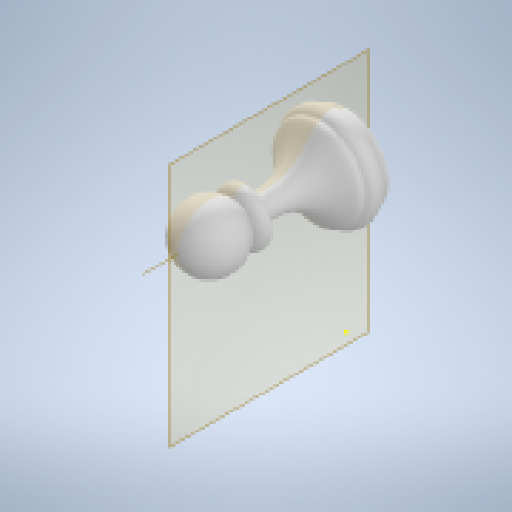
# Autodesk Inventor part: pawn-white-v2
Saved by Autodesk Inventor 2024.1 (Build 281209000, 209)
## iProperties
Created: 2025-08-03
Part Number: pawn-white-v2
Material: Generic
Document SubType Name: Modeling
Designer: iwheard
Density: 1 g/cm^3
Appearance: Default
Author: iwheard
Autodesk Inventor part; units mm, degrees
(part 1 of 2)
ref_plane "XZ Plane" through (0, 0, 0) normal (0, 1, 0) x (-1, 0, 0)
ref_plane "XY Plane" through (0, 0, 0) normal (0, 0, 1) x (1, 0, 0)
sketch "Sketch1" plane through (0, 0, 0) normal (0, 0, 1) x (1, 0, 0)
  circle A0 centre (0, 25.5) radius 3
  circle A1 centre (0, 25.5) radius 5
  point P0 (0, 0)
  dimension "d0" = 10
  constraints: 2 centre point
  measures "d0" diameter of A1
extrude "Extrusion1" add sketch "Sketch1" along normal blind 3
sketch "Sketch3" plane through (0, 25.5, 3) normal (0, 0, 1) x (1, 0, 0)
  circle A0 centre (0, 0) radius 5 projected
  circle A1 centre (0, 0) radius 3 projected
  circle A2 centre (0, 0) radius 7.15
  point P0 (0, -25.5)
  dimension "d6" = 14.3
  constraints: 1 centre point
  measures "d6" diameter of A2
extrude "Extrusion2" add sketch "Sketch3" against normal blind 3 contours A2
sketch "Sketch2" plane through (0, 0, 0) normal (1, 0, 0) x (0, 1, 0)
  line L0 (30.5, 3) -> (20.5, 3) projected
  circle A0 centre (25.5, 23) radius 5.25
  line L1 (30.5, 0) -> (20.5, 0) projected
  line L2 (25.5, 28.25) -> (25.5, 3)
  line L3 (28.7742, 18.8961) -> (28.7225, 18.9815) construction
  line L4 (27.5353, 15.1585) -> (27.5353, 12.8331) construction
  line L5 (27.5353, 12.8331) -> (27.8628, 9.8109) construction
  line L6 (27.8628, 9.8109) -> (30.696, 6.4585) construction
  line L7 (30.696, 6.4585) -> (33.4932, 5.0528) construction
  line L8 (34.1113, 1.8552) -> (32.8751, 0.9289) construction
  line L9 (32.8751, 0.9289) -> (32.65, 0.7147) construction
  spline S0 degree 4 poles (28.7742, 18.8961) (28.7225, 18.9815) (30.0018, 18.4917) (30.1859, 16.8801) (29.2697, 16.5797) (27.9179, 16.8801) (27.9179, 16.1364) (27.5353, 15.1585) (27.5353, 12.8331) (27.8628, 9.8109) (30.696, 6.4585) (33.4932, 5.0528) (32.5369, 4.2802) (33.817, 3.9218) (34.1113, 1.8552) (32.8751, 0.9289) (32.65, 0.7147) knots 0 0 0 0 0 0.002456 0.076412 0.193262 1 2 3 4 5 6 7 7.40272 8 9 9 9 9 9
  line L10 (30.5, 0) -> (30.5, 3) projected
  line L11 (27.9179, 16.1364) -> (27.5353, 15.1585) construction
  line L12 (28.5, 3) -> (28.5, 0) projected
  line L13 (32.65, 3) -> (18.35, 3) projected
  line L14 (32.65, 3) -> (32.65, 0) projected
  line L15 (33.4932, 5.0528) -> (32.5369, 4.2802) construction
  line L16 (32.5369, 4.2802) -> (33.817, 3.9218) construction
  line L17 (33.817, 3.9218) -> (34.1113, 1.8552) construction
  line L18 (27.9179, 16.8801) -> (27.9179, 16.1364) construction
  line L19 (29.2697, 16.5797) -> (27.9179, 16.8801) construction
  line L20 (28.7225, 18.9815) -> (30.0018, 18.4917) construction
  line L21 (30.0018, 18.4917) -> (30.1859, 16.8801) construction
  line L22 (30.1859, 16.8801) -> (29.2697, 16.5797) construction
  point P0 (0, 0)
  point P1 (25.5, 3)
  point P2 (30.5, 0.7117)
  point P3 (28.8281, 18.9396)
  point P4 (25.5, 17.75)
  point P5 (32.65, 0.7147)
  dimension "d3" = 10.5
  dimension "d4" = 23
  constraints: 2 end point, 2 point on circle, 2 vertical alignment, 1 centre point, 1 midpoint, 4 other
  measures "d3" diameter of A0
  measures "d4" distance from line of L1 A0.centre
revolve "Revolution1" add sketch "Sketch2" angle 360 about axis through (0, 25.5, 28.25) along (0, 0, -1) contours L0 L2 A0 S0 L14 L13 | L2 A0 S0 | A0 S0
chamfer "Chamfer1" distance 0.5 angle 45 2 edges at (5.0558, 30.5558, 0.7147) (-5.0558, 20.4442, 0.7147)
sketch "Sketch11" plane through (0, 0, 0) normal (1, 0, 0) x (0, 1, 0)
  line L0 (27.9316, 16.5405) -> (27.8538, 16.3314)
  line L1 (27.8538, 16.3314) -> (28.5086, 16.0877)
  line L2 (28.5086, 16.0877) -> (28.5864, 16.2967)
  line L3 (28.5864, 16.2967) -> (27.9316, 16.5405)
  line L4 (27.837, 16.2536) -> (27.7455, 15.9057)
  line L5 (27.7455, 15.9057) -> (28.4076, 15.7315)
  line L6 (28.4076, 15.7315) -> (28.4991, 16.0794)
  line L7 (28.4991, 16.0794) -> (27.837, 16.2536)
  line L8 (27.7341, 15.8623) -> (27.561, 15.0978)
  line L9 (27.561, 15.0978) -> (28.3711, 14.9144)
  line L10 (28.3711, 14.9144) -> (28.5442, 15.6789)
  line L11 (28.5442, 15.6789) -> (27.7341, 15.8623)
  line L12 (27.5469, 14.9814) -> (27.5027, 14.0719)
  line L13 (27.5027, 14.0719) -> (28.4029, 14.0282)
  line L14 (28.4029, 14.0282) -> (28.4471, 14.9377)
  line L15 (28.4471, 14.9377) -> (27.5469, 14.9814)
  line L16 (27.4909, 13.8281) -> (27.532, 12.6551)
  line L17 (27.532, 12.6551) -> (28.8485, 12.7012)
  line L18 (28.8485, 12.7012) -> (28.8074, 13.8742)
  line L19 (28.8074, 13.8742) -> (27.4909, 13.8281)
  line L20 (27.5561, 12.4959) -> (27.7913, 11.1635)
  line L21 (27.7913, 11.1635) -> (29.3083, 11.4312)
  line L22 (29.3083, 11.4312) -> (29.0732, 12.7637)
  line L23 (29.0732, 12.7637) -> (27.5561, 12.4959)
  line L24 (27.837, 10.9041) -> (28.2953, 9.6805)
  line L25 (28.2953, 9.6805) -> (29.8371, 10.2579)
  line L26 (29.8371, 10.2579) -> (29.3789, 11.4815)
  line L27 (29.3789, 11.4815) -> (27.837, 10.9041)
  line L28 (28.4029, 9.3932) -> (29.3083, 8.0791)
  line L29 (29.3083, 8.0791) -> (30.9089, 9.1819)
  line L30 (30.9089, 9.1819) -> (30.0035, 10.496)
  line L31 (30.0035, 10.496) -> (28.4029, 9.3932)
  line L32 (29.7117, 7.6092) -> (31.4159, 6.0425)
  line L33 (31.4159, 6.0425) -> (33.1005, 7.8751)
  line L34 (33.1005, 7.8751) -> (31.3962, 9.4417)
  line L35 (31.3962, 9.4417) -> (29.7117, 7.6092)
  line L36 (29.7556, 7.5688) -> (32.638, 5.3084)
  line L37 (32.638, 5.3084) -> (33.9032, 6.9217)
  line L38 (33.9032, 6.9217) -> (31.0207, 9.1822)
  line L39 (31.0207, 9.1822) -> (29.7556, 7.5688)
  point P0 (0, 0)
  point P1 (28.3771, 14.9411)
  point P2 (28.2195, 14.9487)
  point P3 (28.6874, 12.6956)
  point P4 (28.8477, 12.7239)
  point P5 (29.1875, 11.4099)
  point P6 (29.3043, 11.4536)
  point P7 (29.4446, 10.1109)
  point P8 (29.8004, 10.356)
  constraints: 80 end point, 20 parallel, 10 perpendicular, 6 point on line
extrude "Extrusion6" cut sketch "Sketch11" along normal mid plane 10 contours L3 L2 L1 L0 | L7 L6 L5 L4 | L11 L10 L15 L9 L8 | L15 L10 L9 | L9 L10 L15 L14 L13 L12 | L19 L18 L23 L17 L16 | L17 L18 L23 L22 L27 L21 L20 | L27 L26 L31 L25 L24 L21 L22 | L31 L30 L29 L28 L25 L26 | L35 L39 L32 | L36 L33 L32 | L39 L35 L38 L33 L36 | L39 L38 L35 | L33 L38 L37 L36 | L35 L34 L33 L38
sketch "Sketch12" plane through (-2.1873, 31.7347, 5.7495) normal (0, 0.6767574, 0.7362061) x (1, 0, 0)
  line L0 (14.163, 8.8077) -> (14.3706, 8.3256)
  line L1 (14.3706, 8.3256) -> (14.8236, 7.8122)
  line L2 (14.8236, 7.8122) -> (15.3364, 7.3493)
  line L3 (15.3364, 7.3493) -> (15.9624, 7.2197)
  line L4 (15.9624, 7.2197) -> (16.3471, 7.1936)
  line L5 (16.3471, 7.1936) -> (16.622, 7.2886)
  line L6 (16.622, 7.2886) -> (17.37, 8.2151)
  line L7 (17.37, 8.2151) -> (17.7786, 8.8333)
  line L8 (17.7786, 8.8333) -> (17.8374, 9.0234)
  line L9 (17.8374, 9.0234) -> (17.7788, 9.151)
  line L10 (17.7788, 9.151) -> (17.2482, 9.2679)
  line L11 (17.2482, 9.2679) -> (16.0645, 9.2846)
  line L12 (16.0645, 9.2846) -> (14.2757, 9.225)
  line L13 (14.2757, 9.225) -> (14.099, 9.0834)
  line L14 (14.099, 9.0834) -> (14.163, 8.8077)
  line L15 (-0.827, 7.7393) -> (0.3726, 6.4109)
  line L16 (0.3726, 6.4109) -> (0.6073, 6.298)
  line L17 (0.6073, 6.298) -> (0.8022, 6.3831)
  line L18 (0.8022, 6.3831) -> (1.0932, 6.7181)
  line L19 (1.0932, 6.7181) -> (1.3226, 7.9284)
  line L20 (1.3226, 7.9284) -> (1.4204, 8.7124)
  line L21 (1.4204, 8.7124) -> (1.2832, 9.1151)
  line L22 (1.2832, 9.1151) -> (0.7585, 9.2634)
  line L23 (0.7585, 9.2634) -> (-0.3067, 9.2846)
  line L24 (-0.3067, 9.2846) -> (-1.3546, 9.2605)
  line L25 (-1.3546, 9.2605) -> (-1.758, 9.0914)
  line L26 (-1.758, 9.0914) -> (-1.5659, 8.6327)
  line L27 (-1.5659, 8.6327) -> (-0.827, 7.7393)
  line L28 (7.9724, 8.1152) -> (8.0582, 7.0436)
  line L29 (8.0582, 7.0436) -> (8.456, 6.5585)
  line L30 (8.456, 6.5585) -> (8.9127, 6.2422)
  line L31 (8.9127, 6.2422) -> (9.411, 6.3517)
  line L32 (9.411, 6.3517) -> (9.7063, 6.4776)
  line L33 (9.7063, 6.4776) -> (9.8794, 6.6817)
  line L34 (9.8794, 6.6817) -> (10.1275, 7.9084)
  line L35 (10.1275, 7.9084) -> (10.231, 8.704)
  line L36 (10.231, 8.704) -> (10.1625, 9.1126)
  line L37 (10.1625, 9.1126) -> (9.8294, 9.2631)
  line L38 (9.8294, 9.2631) -> (9.1388, 9.2846)
  line L39 (9.1388, 9.2846) -> (8.4456, 9.2663)
  line L40 (8.4456, 9.2663) -> (8.093, 9.1384)
  line L41 (8.093, 9.1384) -> (7.9717, 8.7913)
  line L42 (7.9717, 8.7913) -> (7.9724, 8.1152)
  line L43 (5.0826, 8.0719) -> (5.1312, 7.3559)
  line L44 (5.1312, 7.3559) -> (5.3208, 6.9613)
  line L45 (5.3208, 6.9613) -> (5.7267, 6.7901)
  line L46 (5.7267, 6.7901) -> (6.4238, 6.744)
  line L47 (6.4238, 6.744) -> (7.4596, 6.7391)
  line L48 (7.4596, 6.7391) -> (7.7676, 6.8351)
  line L49 (7.7676, 6.8351) -> (7.9267, 7.0799)
  line L50 (7.9267, 7.0799) -> (7.9205, 8.1163)
  line L51 (7.9205, 8.1163) -> (7.8791, 8.7917)
  line L52 (7.8791, 8.7917) -> (7.7156, 9.1386)
  line L53 (7.7156, 9.1386) -> (7.295, 9.2663)
  line L54 (7.295, 9.2663) -> (6.4826, 9.2846)
  line L55 (6.4826, 9.2846) -> (5.6709, 9.2657)
  line L56 (5.6709, 9.2657) -> (5.2544, 9.133)
  line L57 (5.2544, 9.133) -> (5.1021, 8.773)
  line L58 (5.1021, 8.773) -> (5.0826, 8.0719)
  line L59 (2.9046, 7.8131) -> (2.9449, 6.9663)
  line L60 (2.9449, 6.9663) -> (3.0705, 6.5566)
  line L61 (3.0705, 6.5566) -> (3.3825, 6.4694)
  line L62 (3.3825, 6.4694) -> (3.982, 6.5898)
  line L63 (3.982, 6.5898) -> (4.5907, 6.7618)
  line L64 (4.5907, 6.7618) -> (4.9028, 6.9733)
  line L65 (4.9028, 6.9733) -> (5.0167, 7.363)
  line L66 (5.0167, 7.363) -> (5.0308, 8.0695)
  line L67 (5.0308, 8.0695) -> (5.0114, 8.772)
  line L68 (5.0114, 8.772) -> (4.8919, 9.1327)
  line L69 (4.8919, 9.1327) -> (4.5702, 9.2656)
  line L70 (4.5702, 9.2656) -> (3.9448, 9.2846)
  line L71 (3.9448, 9.2846) -> (3.3201, 9.2616)
  line L72 (3.3201, 9.2616) -> (3.0035, 9.1007)
  line L73 (3.0035, 9.1007) -> (2.8975, 8.6638)
  line L74 (2.8975, 8.6638) -> (2.9046, 7.8131)
  line L75 (1.9535, 6.3705) -> (2.6599, 6.2006)
  line L76 (2.6599, 6.2006) -> (2.8227, 6.2422)
  line L77 (2.8227, 6.2422) -> (2.8531, 7.8018)
  line L78 (2.8531, 7.8018) -> (2.7404, 9.0993)
  line L79 (2.7404, 9.0993) -> (2.5551, 9.2614)
  line L80 (2.5551, 9.2614) -> (2.2027, 9.2846)
  line L81 (2.2027, 9.2846) -> (1.8475, 9.2634)
  line L82 (1.8475, 9.2634) -> (1.6429, 9.1153)
  line L83 (1.6429, 9.1153) -> (1.3754, 7.9301)
  line L84 (1.3754, 7.9301) -> (1.2613, 7.1439)
  line L85 (1.2613, 7.1439) -> (1.2835, 6.7193)
  line L86 (1.2835, 6.7193) -> (1.4962, 6.5103)
  line L87 (1.4962, 6.5103) -> (1.9535, 6.3705)
  line L88 (10.7348, 6.2426) -> (11.2015, 6.1065)
  line L89 (11.2015, 6.1065) -> (11.5002, 6.2111)
  line L90 (11.5002, 6.2111) -> (11.7035, 6.6792)
  line L91 (11.7035, 6.6792) -> (11.8841, 7.6335)
  line L92 (11.8841, 7.6335) -> (12.0194, 8.588)
  line L93 (12.0194, 8.588) -> (12.0002, 9.0781)
  line L94 (12.0002, 9.0781) -> (11.7686, 9.2588)
  line L95 (11.7686, 9.2588) -> (11.2666, 9.2846)
  line L96 (11.2666, 9.2846) -> (10.7573, 9.2631)
  line L97 (10.7573, 9.2631) -> (10.4744, 9.1124)
  line L98 (10.4744, 9.1124) -> (10.3158, 8.7035)
  line L99 (10.3158, 8.7035) -> (10.1798, 7.9073)
  line L100 (10.1798, 7.9073) -> (10.0695, 7.1065)
  line L101 (10.0695, 7.1065) -> (10.0905, 6.6662)
  line L102 (10.0905, 6.6662) -> (10.2949, 6.4302)
  line L103 (10.2949, 6.4302) -> (10.7348, 6.2426)
  line L104 (16.9589, 6.5843) -> (17.1578, 6.2745)
  line L105 (17.1578, 6.2745) -> (17.393, 6.1023)
  line L106 (17.393, 6.1023) -> (18.5799, 5.9227)
  line L107 (18.5799, 5.9227) -> (19.3386, 5.8753)
  line L108 (19.3386, 5.8753) -> (19.7282, 6.0278)
  line L109 (19.7282, 6.0278) -> (19.8717, 6.5319)
  line L110 (19.8717, 6.5319) -> (19.8922, 7.539)
  line L111 (19.8922, 7.539) -> (19.879, 8.5482)
  line L112 (19.879, 8.5482) -> (19.7863, 9.0664)
  line L113 (19.7863, 9.0664) -> (19.5345, 9.2573)
  line L114 (19.5345, 9.2573) -> (19.0443, 9.2846)
  line L115 (19.0443, 9.2846) -> (18.542, 9.2677)
  line L116 (18.542, 9.2677) -> (18.2057, 9.1491)
  line L117 (18.2057, 9.1491) -> (17.4233, 8.2007)
  line L118 (17.4233, 8.2007) -> (16.7855, 7.1857)
  line L119 (16.7855, 7.1857) -> (16.7926, 6.909)
  line L120 (16.7926, 6.909) -> (16.9589, 6.5843)
  line L121 (12.0155, 5.7626) -> (12.3735, 5.5954)
  line L122 (12.3735, 5.5954) -> (12.8508, 5.6913)
  line L123 (12.8508, 5.6913) -> (13.1456, 5.7916)
  line L124 (13.1456, 5.7916) -> (13.3441, 5.969)
  line L125 (13.3441, 5.969) -> (13.8139, 7.0741)
  line L126 (13.8139, 7.0741) -> (14.2004, 8.2222)
  line L127 (14.2004, 8.2222) -> (14.1104, 8.8011)
  line L128 (14.1104, 8.8011) -> (13.8533, 9.2243)
  line L129 (13.8533, 9.2243) -> (13.0678, 9.2847)
  line L130 (13.0678, 9.2847) -> (12.5587, 9.2588)
  line L131 (12.5587, 9.2588) -> (12.2711, 9.0777)
  line L132 (12.2711, 9.0777) -> (12.0989, 8.5862)
  line L133 (12.0989, 8.5862) -> (11.9359, 7.6291)
  line L134 (11.9359, 7.6291) -> (11.7519, 6.1542)
  line L135 (11.7519, 6.1542) -> (11.824, 5.9105)
  line L136 (11.824, 5.9105) -> (12.0155, 5.7626)
  line L137 (-3.0143, 6.2965) -> (-2.0806, 5.9141)
  line L138 (-2.0806, 5.9141) -> (-0.8838, 5.8842)
  line L139 (-0.8838, 5.8842) -> (0.2085, 5.9246)
  line L140 (0.2085, 5.9246) -> (0.4112, 6.0344)
  line L141 (0.4112, 6.0344) -> (0.2906, 6.3362)
  line L142 (0.2906, 6.3362) -> (-0.879, 7.7202)
  line L143 (-0.879, 7.7202) -> (-2.1604, 9.0891)
  line L144 (-2.1604, 9.0891) -> (-2.557, 9.2602)
  line L145 (-2.557, 9.2602) -> (-3.0638, 9.2846)
  line L146 (-3.0638, 9.2846) -> (-3.5496, 9.2647)
  line L147 (-3.5496, 9.2647) -> (-3.7991, 9.1254)
  line L148 (-3.7991, 9.1254) -> (-3.891, 8.7474)
  line L149 (-3.891, 8.7474) -> (-3.9041, 8.0111)
  line L150 (-3.9041, 8.0111) -> (-3.8902, 7.268)
  line L151 (-3.8902, 7.268) -> (-3.7929, 6.8417)
  line L152 (-3.7929, 6.8417) -> (-3.5287, 6.5715)
  line L153 (-3.5287, 6.5715) -> (-3.0143, 6.2965)
  line L154 (14.0869, 5.443) -> (14.7153, 5.1287)
  line L155 (14.7153, 5.1287) -> (14.991, 5.2011)
  line L156 (14.991, 5.2011) -> (15.1852, 5.441)
  line L157 (15.1852, 5.441) -> (15.2434, 6.2985)
  line L158 (15.2434, 6.2985) -> (15.2143, 7.2021)
  line L159 (15.2143, 7.2021) -> (14.7979, 7.7641)
  line L160 (14.7979, 7.7641) -> (14.5126, 8.037)
  line L161 (14.5126, 8.037) -> (14.3197, 8.053)
  line L162 (14.3197, 8.053) -> (13.8583, 7.0454)
  line L163 (13.8583, 7.0454) -> (13.604, 6.332)
  line L164 (13.604, 6.332) -> (13.543, 5.9273)
  line L165 (13.543, 5.9273) -> (13.6969, 5.681)
  line L166 (13.6969, 5.681) -> (14.0869, 5.443)
  line L167 (15.7925, 5.2639) -> (16.3143, 5.2456)
  line L168 (16.3143, 5.2456) -> (16.772, 5.6072)
  line L169 (16.772, 5.6072) -> (17.1247, 6.0454)
  line L170 (17.1247, 6.0454) -> (16.9114, 6.563)
  line L171 (16.9114, 6.563) -> (16.5625, 7.0367)
  line L172 (16.5625, 7.0367) -> (15.9668, 7.167)
  line L173 (15.9668, 7.167) -> (15.5981, 7.1944)
  line L174 (15.5981, 7.1944) -> (15.4053, 7.1125)
  line L175 (15.4053, 7.1125) -> (15.2951, 6.2928)
  line L176 (15.2951, 6.2928) -> (15.331, 5.4537)
  line L177 (15.331, 5.4537) -> (15.4852, 5.3259)
  line L178 (15.4852, 5.3259) -> (15.7925, 5.2639)
  line L179 (5.8878, 5.9253) -> (6.4103, 5.2372)
  line L180 (6.4103, 5.2372) -> (6.613, 5.1464)
  line L181 (6.613, 5.1464) -> (6.7926, 5.2488)
  line L182 (6.7926, 5.2488) -> (7.154, 5.9131)
  line L183 (7.154, 5.9131) -> (7.363, 6.3516)
  line L184 (7.363, 6.3516) -> (7.3572, 6.579)
  line L185 (7.3572, 6.579) -> (7.0684, 6.6681)
  line L186 (7.0684, 6.6681) -> (6.4288, 6.692)
  line L187 (6.4288, 6.692) -> (5.7921, 6.6918)
  line L188 (5.7921, 6.6918) -> (5.5235, 6.6119)
  line L189 (5.5235, 6.6119) -> (5.5723, 6.3803)
  line L190 (5.5723, 6.3803) -> (5.8878, 5.9253)
  line L191 (2.8903, 5.3703) -> (2.9648, 4.9353)
  line L192 (2.9648, 4.9353) -> (3.0874, 4.7341)
  line L193 (3.0874, 4.7341) -> (3.3405, 4.7184)
  line L194 (3.3405, 4.7184) -> (3.8066, 4.8396)
  line L195 (3.8066, 4.8396) -> (4.5311, 5.1489)
  line L196 (4.5311, 5.1489) -> (4.8015, 5.9253)
  line L197 (4.8015, 5.9253) -> (4.8979, 6.4153)
  line L198 (4.8979, 6.4153) -> (4.843, 6.6419)
  line L199 (4.843, 6.6419) -> (4.5583, 6.662)
  line L200 (4.5583, 6.662) -> (3.9655, 6.5326)
  line L201 (3.9655, 6.5326) -> (2.8605, 6.2067)
  line L202 (2.8605, 6.2067) -> (2.8903, 5.3703)
  line L203 (7.4043, 4.6682) -> (7.7539, 4.4105)
  line L204 (7.7539, 4.4105) -> (7.9777, 4.3656)
  line L205 (7.9777, 4.3656) -> (8.1723, 4.5703)
  line L206 (8.1723, 4.5703) -> (8.4341, 5.0616)
  line L207 (8.4341, 5.0616) -> (8.7631, 6.0447)
  line L208 (8.7631, 6.0447) -> (8.6783, 6.2761)
  line L209 (8.6783, 6.2761) -> (8.4261, 6.5159)
  line L210 (8.4261, 6.5159) -> (8.0108, 6.8395)
  line L211 (8.0108, 6.8395) -> (7.7928, 6.7898)
  line L212 (7.7928, 6.7898) -> (7.581, 6.5955)
  line L213 (7.581, 6.5955) -> (7.2095, 5.9075)
  line L214 (7.2095, 5.9075) -> (6.9353, 5.1749)
  line L215 (6.9353, 5.1749) -> (7.0677, 4.9514)
  line L216 (7.0677, 4.9514) -> (7.4043, 4.6682)
  line L217 (9.604, 5.1782) -> (10.0069, 4.7567)
  line L218 (10.0069, 4.7567) -> (10.2732, 4.6156)
  line L219 (10.2732, 4.6156) -> (10.5217, 4.7544)
  line L220 (10.5217, 4.7544) -> (10.8711, 5.1727)
  line L221 (10.8711, 5.1727) -> (11.198, 5.6071)
  line L222 (11.198, 5.6071) -> (11.289, 5.8592)
  line L223 (11.289, 5.8592) -> (11.1278, 6.025)
  line L224 (11.1278, 6.025) -> (10.6982, 6.201)
  line L225 (10.6982, 6.201) -> (9.9707, 6.4273)
  line L226 (9.9707, 6.4273) -> (9.4326, 6.3044)
  line L227 (9.4326, 6.3044) -> (9.1486, 6.0747)
  line L228 (9.1486, 6.0747) -> (9.0717, 5.8809)
  line L229 (9.0717, 5.8809) -> (9.604, 5.1782)
  line L230 (0.458, 5.1525) -> (0.5521, 4.4772)
  line L231 (0.5521, 4.4772) -> (0.8637, 4.1335)
  line L232 (0.8637, 4.1335) -> (1.3862, 3.8361)
  line L233 (1.3862, 3.8361) -> (2.2517, 4.2176)
  line L234 (2.2517, 4.2176) -> (2.8433, 4.6534)
  line L235 (2.8433, 4.6534) -> (2.8391, 5.3618)
  line L236 (2.8391, 5.3618) -> (2.6483, 6.0473)
  line L237 (2.6483, 6.0473) -> (1.9335, 6.3221)
  line L238 (1.9335, 6.3221) -> (1.1933, 6.4786)
  line L239 (1.1933, 6.4786) -> (0.8239, 6.3355)
  line L240 (0.8239, 6.3355) -> (0.4582, 6.0127)
  line L241 (0.4582, 6.0127) -> (0.458, 5.1525)
  line L242 (0.458, 5.1525) -> (0.458, 5.1525)
  line L243 (5.0895, 4.6461) -> (5.5237, 4.3399)
  line L244 (5.5237, 4.3399) -> (5.9694, 4.6734)
  line L245 (5.9694, 4.6734) -> (6.2189, 4.9405)
  line L246 (6.2189, 4.9405) -> (6.2876, 5.159)
  line L247 (6.2876, 5.159) -> (5.8298, 5.9167)
  line L248 (5.8298, 5.9167) -> (5.3784, 6.4144)
  line L249 (5.3784, 6.4144) -> (5.1264, 6.5817)
  line L250 (5.1264, 6.5817) -> (4.9827, 6.4199)
  line L251 (4.9827, 6.4199) -> (4.8557, 5.9301)
  line L252 (4.8557, 5.9301) -> (4.736, 5.1162)
  line L253 (4.736, 5.1162) -> (5.0895, 4.6461)
  line L254 (-1.4752, 4.9122) -> (-0.8611, 4.1568)
  line L255 (-0.8611, 4.1568) -> (-0.597, 4.1198)
  line L256 (-0.597, 4.1198) -> (-0.2026, 4.2238)
  line L257 (-0.2026, 4.2238) -> (0.373, 4.4918)
  line L258 (0.373, 4.4918) -> (0.4066, 5.1444)
  line L259 (0.4066, 5.1444) -> (0.3548, 5.5582)
  line L260 (0.3548, 5.5582) -> (0.205, 5.7679)
  line L261 (0.205, 5.7679) -> (-0.8661, 5.8328)
  line L262 (-0.8661, 5.8328) -> (-1.5595, 5.8025)
  line L263 (-1.5595, 5.8025) -> (-1.8541, 5.6965)
  line L264 (-1.8541, 5.6965) -> (-1.807, 5.4285)
  line L265 (-1.807, 5.4285) -> (-1.4752, 4.9122)
  line L266 (16.6019, 4.5771) -> (16.7631, 4.2509)
  line L267 (16.7631, 4.2509) -> (17.0005, 4.1094)
  line L268 (17.0005, 4.1094) -> (18.3658, 4.2621)
  line L269 (18.3658, 4.2621) -> (19.7014, 4.5627)
  line L270 (19.7014, 4.5627) -> (19.8684, 4.7722)
  line L271 (19.8684, 4.7722) -> (19.8923, 5.1298)
  line L272 (19.8923, 5.1298) -> (19.8717, 5.4854)
  line L273 (19.8717, 5.4854) -> (19.7278, 5.6811)
  line L274 (19.7278, 5.6811) -> (18.5766, 5.8709)
  line L275 (18.5766, 5.8709) -> (17.3694, 5.931)
  line L276 (17.3694, 5.931) -> (17.0925, 5.8187)
  line L277 (17.0925, 5.8187) -> (16.8127, 5.5743)
  line L278 (16.8127, 5.5743) -> (16.4501, 5.1301)
  line L279 (16.4501, 5.1301) -> (16.6019, 4.5771)
  line L280 (8.4766, 3.7997) -> (8.934, 3.552)
  line L281 (8.934, 3.552) -> (9.545, 3.6089)
  line L282 (9.545, 3.6089) -> (10.1069, 3.7446)
  line L283 (10.1069, 3.7446) -> (10.2205, 4.0484)
  line L284 (10.2205, 4.0484) -> (10.1698, 4.4319)
  line L285 (10.1698, 4.4319) -> (9.5812, 5.1262)
  line L286 (9.5812, 5.1262) -> (9.1823, 5.5441)
  line L287 (9.1823, 5.5441) -> (8.9333, 5.6717)
  line L288 (8.9333, 5.6717) -> (8.7301, 5.4985)
  line L289 (8.7301, 5.4985) -> (8.4681, 5.0139)
  line L290 (8.4681, 5.0139) -> (8.1516, 4.1754)
  line L291 (8.1516, 4.1754) -> (8.2335, 3.9866)
  line L292 (8.2335, 3.9866) -> (8.4766, 3.7997)
  line L293 (12.4477, 4.7273) -> (12.6096, 4.0131)
  line L294 (12.6096, 4.0131) -> (13.3216, 3.6758)
  line L295 (13.3216, 3.6758) -> (14.0451, 3.4443)
  line L296 (14.0451, 3.4443) -> (14.2875, 3.4715)
  line L297 (14.2875, 3.4715) -> (14.4479, 3.6254)
  line L298 (14.4479, 3.6254) -> (14.5978, 4.2811)
  line L299 (14.5978, 4.2811) -> (14.641, 4.9757)
  line L300 (14.641, 4.9757) -> (14.0552, 5.4012)
  line L301 (14.0552, 5.4012) -> (13.3891, 5.717)
  line L302 (13.3891, 5.717) -> (12.8709, 5.6431)
  line L303 (12.8709, 5.6431) -> (12.4479, 5.4246)
  line L304 (12.4479, 5.4246) -> (12.4477, 4.7273)
  line L305 (10.3448, 3.6081) -> (11.1727, 3.4681)
  line L306 (11.1727, 3.4681) -> (11.835, 3.4626)
  line L307 (11.835, 3.4626) -> (12.1775, 3.6834)
  line L308 (12.1775, 3.6834) -> (12.4217, 4.0074)
  line L309 (12.4217, 4.0074) -> (12.3958, 4.7251)
  line L310 (12.3958, 4.7251) -> (12.2913, 5.4369)
  line L311 (12.2913, 5.4369) -> (11.9846, 5.7207)
  line L312 (11.9846, 5.7207) -> (11.7032, 5.8153)
  line L313 (11.7032, 5.8153) -> (11.4977, 5.7865)
  line L314 (11.4977, 5.7865) -> (10.9127, 5.1418)
  line L315 (10.9127, 5.1418) -> (10.3816, 4.4319)
  line L316 (10.3816, 4.4319) -> (10.2719, 4.0418)
  line L317 (10.2719, 4.0418) -> (10.2514, 3.735)
  line L318 (10.2514, 3.735) -> (10.3448, 3.6081)
  line L319 (-2.7436, 3.2905) -> (-1.6862, 3.2268)
  line L320 (-1.6862, 3.2268) -> (-1.4595, 3.3359)
  line L321 (-1.4595, 3.3359) -> (-1.2473, 3.5745)
  line L322 (-1.2473, 3.5745) -> (-1.0628, 3.8293)
  line L323 (-1.0628, 3.8293) -> (-1.0307, 4.0523)
  line L324 (-1.0307, 4.0523) -> (-1.5296, 4.8999)
  line L325 (-1.5296, 4.8999) -> (-2.1803, 5.7499)
  line L326 (-2.1803, 5.7499) -> (-3.026, 6.2445)
  line L327 (-3.026, 6.2445) -> (-3.5337, 6.4707)
  line L328 (-3.5337, 6.4707) -> (-3.7944, 6.4218)
  line L329 (-3.7944, 6.4218) -> (-3.8904, 5.986)
  line L330 (-3.8904, 5.986) -> (-3.9041, 5.0513)
  line L331 (-3.9041, 5.0513) -> (-3.886, 4.1077)
  line L332 (-3.886, 4.1077) -> (-3.7591, 3.6097)
  line L333 (-3.7591, 3.6097) -> (-3.4145, 3.3924)
  line L334 (-3.4145, 3.3924) -> (-2.7436, 3.2905)
  line L335 (15.33, 3.0883) -> (15.821, 2.8441)
  line L336 (15.821, 2.8441) -> (16.1155, 2.7935)
  line L337 (16.1155, 2.7935) -> (16.3099, 2.9494)
  line L338 (16.3099, 2.9494) -> (16.5006, 3.3248)
  line L339 (16.5006, 3.3248) -> (16.7283, 3.9679)
  line L340 (16.7283, 3.9679) -> (16.5552, 4.5543)
  line L341 (16.5552, 4.5543) -> (16.278, 5.0695)
  line L342 (16.278, 5.0695) -> (15.7771, 5.2138)
  line L343 (15.7771, 5.2138) -> (15.2787, 5.2686)
  line L344 (15.2787, 5.2686) -> (15.0186, 5.1572)
  line L345 (15.0186, 5.1572) -> (14.8072, 4.943)
  line L346 (14.8072, 4.943) -> (14.6499, 4.2776)
  line L347 (14.6499, 4.2776) -> (14.5771, 3.8425)
  line L348 (14.5771, 3.8425) -> (14.6237, 3.5736)
  line L349 (14.6237, 3.5736) -> (15.33, 3.0883)
  line L350 (3.8163, 3.5254) -> (4.5452, 2.6316)
  line L351 (4.5452, 2.6316) -> (4.7642, 2.5585)
  line L352 (4.7642, 2.5585) -> (5.0393, 2.6214)
  line L353 (5.0393, 2.6214) -> (5.4375, 2.8306)
  line L354 (5.4375, 2.8306) -> (5.4952, 3.4723)
  line L355 (5.4952, 3.4723) -> (5.4414, 4.149)
  line L356 (5.4414, 4.149) -> (5.0588, 4.6037)
  line L357 (5.0588, 4.6037) -> (4.5778, 4.9407)
  line L358 (4.5778, 4.9407) -> (3.8349, 4.7938)
  line L359 (3.8349, 4.7938) -> (3.3922, 4.646)
  line L360 (3.3922, 4.646) -> (3.2427, 4.4647)
  line L361 (3.2427, 4.4647) -> (3.3846, 4.1307)
  line L362 (3.3846, 4.1307) -> (3.8163, 3.5254)
  line L363 (6.0419, 2.7871) -> (6.551, 2.8995)
  line L364 (6.551, 2.8995) -> (7.2557, 3.4588)
  line L365 (7.2557, 3.4588) -> (7.6664, 3.8629)
  line L366 (7.6664, 3.8629) -> (7.8159, 4.1189)
  line L367 (7.8159, 4.1189) -> (7.7154, 4.3363)
  line L368 (7.7154, 4.3363) -> (7.3763, 4.6242)
  line L369 (7.3763, 4.6242) -> (6.8267, 5.0426)
  line L370 (6.8267, 5.0426) -> (6.6163, 5.0946)
  line L371 (6.6163, 5.0946) -> (6.4244, 5.0305)
  line L372 (6.4244, 5.0305) -> (6.0052, 4.6359)
  line L373 (6.0052, 4.6359) -> (5.605, 4.1531)
  line L374 (5.605, 4.1531) -> (5.5471, 3.4716)
  line L375 (5.5471, 3.4716) -> (5.6227, 2.8442)
  line L376 (5.6227, 2.8442) -> (6.0419, 2.7871)
  line L377 (17.778, 2.518) -> (19.1394, 2.3894)
  line L378 (19.1394, 2.3894) -> (19.5916, 2.4439)
  line L379 (19.5916, 2.4439) -> (19.7654, 2.5082)
  line L380 (19.7654, 2.5082) -> (19.8547, 2.6394)
  line L381 (19.8547, 2.6394) -> (19.8922, 3.4974)
  line L382 (19.8922, 3.4974) -> (19.8684, 4.0532)
  line L383 (19.8684, 4.0532) -> (19.7016, 4.3126)
  line L384 (19.7016, 4.3126) -> (19.2487, 4.3425)
  line L385 (19.2487, 4.3425) -> (18.3668, 4.2097)
  line L386 (18.3668, 4.2097) -> (16.996, 3.9059)
  line L387 (16.996, 3.9059) -> (16.7436, 3.6884)
  line L388 (16.7436, 3.6884) -> (16.5532, 3.3154)
  line L389 (16.5532, 3.3154) -> (16.4102, 2.9438)
  line L390 (16.4102, 2.9438) -> (16.4902, 2.7369)
  line L391 (16.4902, 2.7369) -> (17.778, 2.518)
  line L392 (2.1988, 2.8532) -> (2.8031, 2.0378)
  line L393 (2.8031, 2.0378) -> (3.0659, 1.9491)
  line L394 (3.0659, 1.9491) -> (3.4603, 1.9615)
  line L395 (3.4603, 1.9615) -> (4.069, 2.0305)
  line L396 (4.069, 2.0305) -> (4.3335, 2.2323)
  line L397 (4.3335, 2.2323) -> (4.4412, 2.3781)
  line L398 (4.4412, 2.3781) -> (4.4178, 2.5596)
  line L399 (4.4178, 2.5596) -> (3.7649, 3.5078)
  line L400 (3.7649, 3.5078) -> (3.2963, 4.1132)
  line L401 (3.2963, 4.1132) -> (2.9863, 4.3849)
  line L402 (2.9863, 4.3849) -> (2.6964, 4.3858)
  line L403 (2.6964, 4.3858) -> (2.2881, 4.1786)
  line L404 (2.2881, 4.1786) -> (1.9016, 3.9403)
  line L405 (1.9016, 3.9403) -> (1.7634, 3.7228)
  line L406 (1.7634, 3.7228) -> (1.8653, 3.4019)
  line L407 (1.8653, 3.4019) -> (2.1988, 2.8532)
  line L408 (-1.3052, 2.6747) -> (-1.0024, 2.2793)
  line L409 (-1.0024, 2.2793) -> (-0.2975, 2.2301)
  line L410 (-0.2975, 2.2301) -> (0.4214, 2.3358)
  line L411 (0.4214, 2.3358) -> (0.8223, 3.0254)
  line L412 (0.8223, 3.0254) -> (1.0838, 3.7493)
  line L413 (1.0838, 3.7493) -> (1.0202, 3.9197)
  line L414 (1.0202, 3.9197) -> (0.8276, 4.0962)
  line L415 (0.8276, 4.0962) -> (0.4436, 4.3188)
  line L416 (0.4436, 4.3188) -> (-0.1895, 4.1735)
  line L417 (-0.1895, 4.1735) -> (-0.822, 3.9403)
  line L418 (-0.822, 3.9403) -> (-1.2025, 3.5474)
  line L419 (-1.2025, 3.5474) -> (-1.4693, 3.1236)
  line L420 (-1.4693, 3.1236) -> (-1.3052, 2.6747)
  line L421 (12.1359, 2.3044) -> (12.3347, 1.3421)
  line L422 (12.3347, 1.3421) -> (12.465, 1.1127)
  line L423 (12.465, 1.1127) -> (12.6195, 1.0341)
  line L424 (12.6195, 1.0341) -> (12.9413, 1.1407)
  line L425 (12.9413, 1.1407) -> (13.2974, 1.391)
  line L426 (13.2974, 1.391) -> (13.6919, 2.3179)
  line L427 (13.6919, 2.3179) -> (13.9112, 2.9232)
  line L428 (13.9112, 2.9232) -> (13.9429, 3.2618)
  line L429 (13.9429, 3.2618) -> (13.7503, 3.4562)
  line L430 (13.7503, 3.4562) -> (13.2961, 3.6297)
  line L431 (13.2961, 3.6297) -> (12.5633, 3.8357)
  line L432 (12.5633, 3.8357) -> (12.2127, 3.6453)
  line L433 (12.2127, 3.6453) -> (12.0501, 3.4801)
  line L434 (12.0501, 3.4801) -> (11.9879, 3.2854)
  line L435 (11.9879, 3.2854) -> (12.1359, 2.3044)
  line L436 (7.1734, 2.2974) -> (7.7565, 1.8691)
  line L437 (7.7565, 1.8691) -> (8.2115, 1.887)
  line L438 (8.2115, 1.887) -> (8.6053, 2.0605)
  line L439 (8.6053, 2.0605) -> (8.7596, 2.7206)
  line L440 (8.7596, 2.7206) -> (8.8067, 3.4059)
  line L441 (8.8067, 3.4059) -> (8.4487, 3.756)
  line L442 (8.4487, 3.756) -> (8.1913, 3.9163)
  line L443 (8.1913, 3.9163) -> (7.9855, 3.9353)
  line L444 (7.9855, 3.9353) -> (7.2961, 3.4252)
  line L445 (7.2961, 3.4252) -> (6.8852, 3.056)
  line L446 (6.8852, 3.056) -> (6.7354, 2.8154)
  line L447 (6.7354, 2.8154) -> (6.8354, 2.5978)
  line L448 (6.8354, 2.5978) -> (7.1734, 2.2974)
  line L449 (9.0558, 1.6373) -> (9.614, 1.2706)
  line L450 (9.614, 1.2706) -> (9.8243, 1.2614)
  line L451 (9.8243, 1.2614) -> (10.107, 1.4176)
  line L452 (10.107, 1.4176) -> (10.366, 1.6954)
  line L453 (10.366, 1.6954) -> (10.4112, 2.5377)
  line L454 (10.4112, 2.5377) -> (10.4057, 3.3692)
  line L455 (10.4057, 3.3692) -> (10.3091, 3.5705)
  line L456 (10.3091, 3.5705) -> (10.1319, 3.6413)
  line L457 (10.1319, 3.6413) -> (9.5612, 3.5591)
  line L458 (9.5612, 3.5591) -> (8.9902, 3.3722)
  line L459 (8.9902, 3.3722) -> (8.8104, 2.7094)
  line L460 (8.8104, 2.7094) -> (8.7551, 2.0189)
  line L461 (8.7551, 2.0189) -> (9.0558, 1.6373)
  line L462 (11.3715, 1.4237) -> (11.899, 1.3339)
  line L463 (11.899, 1.3339) -> (12.1489, 1.3959)
  line L464 (12.1489, 1.3959) -> (12.1879, 1.6926)
  line L465 (12.1879, 1.6926) -> (12.0827, 2.3066)
  line L466 (12.0827, 2.3066) -> (11.8141, 3.2456)
  line L467 (11.8141, 3.2456) -> (11.5831, 3.3749)
  line L468 (11.5831, 3.3749) -> (11.1742, 3.4161)
  line L469 (11.1742, 3.4161) -> (10.7684, 3.4261)
  line L470 (10.7684, 3.4261) -> (10.559, 3.3375)
  line L471 (10.559, 3.3375) -> (10.463, 2.5332)
  line L472 (10.463, 2.5332) -> (10.4719, 1.9954)
  line L473 (10.4719, 1.9954) -> (10.5695, 1.7006)
  line L474 (10.5695, 1.7006) -> (10.8409, 1.5447)
  line L475 (10.8409, 1.5447) -> (11.3715, 1.4237)
  line L476 (0.6764, 1.8783) -> (0.905, 1.578)
  line L477 (0.905, 1.578) -> (1.5663, 1.4839)
  line L478 (1.5663, 1.4839) -> (2.2361, 1.4609)
  line L479 (2.2361, 1.4609) -> (2.5238, 1.6576)
  line L480 (2.5238, 1.6576) -> (2.644, 1.8073)
  line L481 (2.644, 1.8073) -> (2.6451, 1.9796)
  line L482 (2.6451, 1.9796) -> (2.15, 2.8333)
  line L483 (2.15, 2.8333) -> (1.6061, 3.659)
  line L484 (1.6061, 3.659) -> (1.3852, 3.7843)
  line L485 (1.3852, 3.7843) -> (1.1954, 3.693)
  line L486 (1.1954, 3.693) -> (0.8691, 3.003)
  line L487 (0.8691, 3.003) -> (0.5831, 2.27)
  line L488 (0.5831, 2.27) -> (0.6764, 1.8783)
  line L489 (14.1034, 1.0582) -> (14.5514, 0.9461)
  line L490 (14.5514, 0.9461) -> (14.8458, 0.9762)
  line L491 (14.8458, 0.9762) -> (15.4952, 1.7064)
  line L492 (15.4952, 1.7064) -> (15.8504, 2.227)
  line L493 (15.8504, 2.227) -> (15.9486, 2.54)
  line L494 (15.9486, 2.54) -> (15.7718, 2.7707)
  line L495 (15.7718, 2.7707) -> (15.3016, 3.0447)
  line L496 (15.3016, 3.0447) -> (14.5547, 3.4296)
  line L497 (14.5547, 3.4296) -> (14.309, 3.4243)
  line L498 (14.309, 3.4243) -> (14.1169, 3.2329)
  line L499 (14.1169, 3.2329) -> (13.7461, 2.3148)
  line L500 (13.7461, 2.3148) -> (13.5263, 1.7105)
  line L501 (13.5263, 1.7105) -> (13.4903, 1.3782)
  line L502 (13.4903, 1.3782) -> (13.6714, 1.2)
  line L503 (13.6714, 1.2) -> (14.1034, 1.0582)
  line L504 (-2.7368, 0.4945) -> (-2.0583, 0.5354)
  line L505 (-2.0583, 0.5354) -> (-1.6868, 0.6401)
  line L506 (-1.6868, 0.6401) -> (-1.4913, 0.8902)
  line L507 (-1.4913, 0.8902) -> (-1.3411, 1.3678)
  line L508 (-1.3411, 1.3678) -> (-1.171, 2.1466)
  line L509 (-1.171, 2.1466) -> (-1.3506, 2.6497)
  line L510 (-1.3506, 2.6497) -> (-1.5062, 2.9159)
  line L511 (-1.5062, 2.9159) -> (-1.7035, 3.0661)
  line L512 (-1.7035, 3.0661) -> (-2.7463, 3.2386)
  line L513 (-2.7463, 3.2386) -> (-3.4157, 3.292)
  line L514 (-3.4157, 3.292) -> (-3.7594, 3.1712)
  line L515 (-3.7594, 3.1712) -> (-3.8861, 2.7515)
  line L516 (-3.8861, 2.7515) -> (-3.9041, 1.9082)
  line L517 (-3.9041, 1.9082) -> (-3.8859, 1.0636)
  line L518 (-3.8859, 1.0636) -> (-3.7582, 0.6348)
  line L519 (-3.7582, 0.6348) -> (-3.4117, 0.4892)
  line L520 (-3.4117, 0.4892) -> (-2.7368, 0.4945)
  line L521 (16.7064, 1.5907) -> (17.0361, 1.0391)
  line L522 (17.0361, 1.0391) -> (17.3213, 0.8411)
  line L523 (17.3213, 0.8411) -> (17.6889, 0.9858)
  line L524 (17.6889, 0.9858) -> (18.2661, 1.462)
  line L525 (18.2661, 1.462) -> (18.8009, 1.9564)
  line L526 (18.8009, 1.9564) -> (18.9236, 2.2263)
  line L527 (18.9236, 2.2263) -> (18.5842, 2.3662)
  line L528 (18.5842, 2.3662) -> (17.7326, 2.4706)
  line L529 (17.7326, 2.4706) -> (16.8436, 2.511)
  line L530 (16.8436, 2.511) -> (16.4404, 2.4328)
  line L531 (16.4404, 2.4328) -> (16.4267, 2.1535)
  line L532 (16.4267, 2.1535) -> (16.7064, 1.5907)
  line L533 (5.9812, 1.6476) -> (6.3822, 0.7443)
  line L534 (6.3822, 0.7443) -> (6.5793, 0.6702)
  line L535 (6.5793, 0.6702) -> (6.8872, 0.7337)
  line L536 (6.8872, 0.7337) -> (7.3649, 0.9101)
  line L537 (7.3649, 0.9101) -> (7.5749, 1.3153)
  line L538 (7.5749, 1.3153) -> (7.6433, 1.7665)
  line L539 (7.6433, 1.7665) -> (7.1303, 2.2658)
  line L540 (7.1303, 2.2658) -> (6.539, 2.7051)
  line L541 (6.539, 2.7051) -> (6.0589, 2.7365)
  line L542 (6.0589, 2.7365) -> (5.7982, 2.6988)
  line L543 (5.7982, 2.6988) -> (5.7031, 2.5728)
  line L544 (5.7031, 2.5728) -> (5.9812, 1.6476)
  line L545 (-0.5316, 0.5882) -> (0.333, 0.7127)
  line L546 (0.333, 0.7127) -> (0.6092, 1.0942)
  line L547 (0.6092, 1.0942) -> (0.7456, 1.5072)
  line L548 (0.7456, 1.5072) -> (0.6312, 1.8526)
  line L549 (0.6312, 1.8526) -> (0.3983, 2.1439)
  line L550 (0.3983, 2.1439) -> (-0.2951, 2.1782)
  line L551 (-0.2951, 2.1782) -> (-0.7439, 2.1605)
  line L552 (-0.7439, 2.1605) -> (-0.9974, 2.0682)
  line L553 (-0.9974, 2.0682) -> (-1.2926, 1.3486)
  line L554 (-1.2926, 1.3486) -> (-1.3941, 0.863)
  line L555 (-1.3941, 0.863) -> (-1.3486, 0.6219)
  line L556 (-1.3486, 0.6219) -> (-1.0849, 0.5541)
  line L557 (-1.0849, 0.5541) -> (-0.5316, 0.5882)
  line L558 (14.9905, 0.6348) -> (15.1436, 0.4452)
  line L559 (15.1436, 0.4452) -> (15.6835, 0.1598)
  line L560 (15.6835, 0.1598) -> (16.2682, -0.0578)
  line L561 (16.2682, -0.0578) -> (16.7356, 0.2272)
  line L562 (16.7356, 0.2272) -> (16.9864, 0.4553)
  line L563 (16.9864, 0.4553) -> (17.0628, 0.6697)
  line L564 (17.0628, 0.6697) -> (16.6669, 1.5547)
  line L565 (16.6669, 1.5547) -> (16.3587, 2.0957)
  line L566 (16.3587, 2.0957) -> (16.1371, 2.2871)
  line L567 (16.1371, 2.2871) -> (15.8952, 2.1389)
  line L568 (15.8952, 2.1389) -> (15.5262, 1.661)
  line L569 (15.5262, 1.661) -> (14.991, 0.8934)
  line L570 (14.991, 0.8934) -> (14.9905, 0.6348)
  line L571 (7.8444, 0.43) -> (8.0761, 0.1937)
  line L572 (8.0761, 0.1937) -> (8.2527, 0.137)
  line L573 (8.2527, 0.137) -> (8.7986, 0.6426)
  line L574 (8.7986, 0.6426) -> (9.2521, 1.242)
  line L575 (9.2521, 1.242) -> (9.2093, 1.4081)
  line L576 (9.2093, 1.4081) -> (9.0139, 1.6054)
  line L577 (9.0139, 1.6054) -> (8.6502, 1.8774)
  line L578 (8.6502, 1.8774) -> (8.2253, 1.8369)
  line L579 (8.2253, 1.8369) -> (7.8239, 1.7004)
  line L580 (7.8239, 1.7004) -> (7.6246, 1.3002)
  line L581 (7.6246, 1.3002) -> (7.5278, 0.8583)
  line L582 (7.5278, 0.8583) -> (7.8444, 0.43)
  line L583 (4.257, 1.1431) -> (4.4068, 0.3813)
  line L584 (4.4068, 0.3813) -> (4.9056, 0.0361)
  line L585 (4.9056, 0.0361) -> (5.4295, -0.1903)
  line L586 (5.4295, -0.1903) -> (5.7546, -0.1211)
  line L587 (5.7546, -0.1211) -> (6.0272, 0.0182)
  line L588 (6.0272, 0.0182) -> (6.1836, 0.2816)
  line L589 (6.1836, 0.2816) -> (6.2548, 0.6639)
  line L590 (6.2548, 0.6639) -> (5.9308, 1.6344)
  line L591 (5.9308, 1.6344) -> (5.5123, 2.5596)
  line L592 (5.5123, 2.5596) -> (5.3292, 2.6359)
  line L593 (5.3292, 2.6359) -> (5.0537, 2.5717)
  line L594 (5.0537, 2.5717) -> (4.6202, 2.4204)
  line L595 (4.6202, 2.4204) -> (4.377, 2.2029)
  line L596 (4.377, 2.2029) -> (4.2034, 1.899)
  line L597 (4.2034, 1.899) -> (4.257, 1.1431)
  line L598 (0.7818, 0.1397) -> (1.1217, -0.3102)
  line L599 (1.1217, -0.3102) -> (1.6774, -0.4127)
  line L600 (1.6774, -0.4127) -> (2.0195, -0.4243)
  line L601 (2.0195, -0.4243) -> (2.196, -0.3374)
  line L602 (2.196, -0.3374) -> (2.2764, 0.458)
  line L603 (2.2764, 0.458) -> (2.1922, 1.2665)
  line L604 (2.1922, 1.2665) -> (1.9775, 1.3841)
  line L605 (1.9775, 1.3841) -> (1.5581, 1.4326)
  line L606 (1.5581, 1.4326) -> (0.9009, 1.4315)
  line L607 (0.9009, 1.4315) -> (0.6551, 1.0695)
  line L608 (0.6551, 1.0695) -> (0.538, 0.6368)
  line L609 (0.538, 0.6368) -> (0.7818, 0.1397)
  line L610 (2.5628, -0.6798) -> (2.7144, -0.7897)
  line L611 (2.7144, -0.7897) -> (2.8679, -0.7857)
  line L612 (2.8679, -0.7857) -> (3.551, -0.2899)
  line L613 (3.551, -0.2899) -> (4.1924, 0.3348)
  line L614 (4.1924, 0.3348) -> (4.2062, 1.131)
  line L615 (4.2062, 1.131) -> (4.0441, 1.8468)
  line L616 (4.0441, 1.8468) -> (3.8377, 1.9231)
  line L617 (3.8377, 1.9231) -> (3.4539, 1.9091)
  line L618 (3.4539, 1.9091) -> (2.8466, 1.8386)
  line L619 (2.8466, 1.8386) -> (2.5641, 1.6247)
  line L620 (2.5641, 1.6247) -> (2.3634, 1.3003)
  line L621 (2.3634, 1.3003) -> (2.3283, 0.4567)
  line L622 (2.3283, 0.4567) -> (2.3519, -0.383)
  line L623 (2.3519, -0.383) -> (2.5628, -0.6798)
  line L624 (18.6199, -0.5657) -> (19.3553, -1.1979)
  line L625 (19.3553, -1.1979) -> (19.7329, -1.3101)
  line L626 (19.7329, -1.3101) -> (19.8719, -0.8138)
  line L627 (19.8719, -0.8138) -> (19.8918, 0.3798)
  line L628 (19.8918, 0.3798) -> (19.855, 2.2032)
  line L629 (19.855, 2.2032) -> (19.768, 2.4077)
  line L630 (19.768, 2.4077) -> (19.5985, 2.3925)
  line L631 (19.5985, 2.3925) -> (19.2196, 2.2121)
  line L632 (19.2196, 2.2121) -> (18.3267, 1.447)
  line L633 (18.3267, 1.447) -> (17.7808, 0.9303)
  line L634 (17.7808, 0.9303) -> (17.6294, 0.5484)
  line L635 (17.6294, 0.5484) -> (17.8999, 0.1126)
  line L636 (17.8999, 0.1126) -> (18.6199, -0.5657)
  line L637 (10.0888, 0.1562) -> (10.2458, -0.4294)
  line L638 (10.2458, -0.4294) -> (10.4379, -0.6357)
  line L639 (10.4379, -0.6357) -> (10.791, -0.4724)
  line L640 (10.791, -0.4724) -> (11.431, 0.0506)
  line L641 (11.431, 0.0506) -> (12.3799, 0.879)
  line L642 (12.3799, 0.879) -> (12.4675, 1.0106)
  line L643 (12.4675, 1.0106) -> (12.4207, 1.0828)
  line L644 (12.4207, 1.0828) -> (11.3713, 1.3709)
  line L645 (11.3713, 1.3709) -> (10.5132, 1.513)
  line L646 (10.5132, 1.513) -> (10.1397, 1.3769)
  line L647 (10.1397, 1.3769) -> (9.9742, 1.2551)
  line L648 (9.9742, 1.2551) -> (9.9137, 1.0874)
  line L649 (9.9137, 1.0874) -> (10.0888, 0.1562)
  line L650 (8.2983, -0.9661) -> (8.3685, -1.8489)
  line L651 (8.3685, -1.8489) -> (8.6081, -2.4971)
  line L652 (8.6081, -2.4971) -> (8.8915, -3.03)
  line L653 (8.8915, -3.03) -> (9.2678, -3.1061)
  line L654 (9.2678, -3.1061) -> (9.4992, -3.089)
  line L655 (9.4992, -3.089) -> (9.6499, -2.9699)
  line L656 (9.6499, -2.9699) -> (9.9739, -2.0172)
  line L657 (9.9739, -2.0172) -> (10.2182, -0.9325)
  line L658 (10.2182, -0.9325) -> (10.0421, 0.1278)
  line L659 (10.0421, 0.1278) -> (9.8029, 1.0566)
  line L660 (9.8029, 1.0566) -> (9.6047, 1.2196)
  line L661 (9.6047, 1.2196) -> (9.3649, 1.1694)
  line L662 (9.3649, 1.1694) -> (8.8348, 0.6054)
  line L663 (8.8348, 0.6054) -> (8.3339, -0.0783)
  line L664 (8.3339, -0.0783) -> (8.2983, -0.9661)
  line L665 (7.1918, -0.9262) -> (8.1441, -1.6108)
  line L666 (8.1441, -1.6108) -> (8.2517, -1.4445)
  line L667 (8.2517, -1.4445) -> (8.2452, -0.941)
  line L668 (8.2452, -0.941) -> (8.1606, -0.1031)
  line L669 (8.1606, -0.1031) -> (7.8125, 0.388)
  line L670 (7.8125, 0.388) -> (7.4037, 0.7497)
  line L671 (7.4037, 0.7497) -> (6.8937, 0.6818)
  line L672 (6.8937, 0.6818) -> (6.4159, 0.5249)
  line L673 (6.4159, 0.5249) -> (6.2323, 0.2633)
  line L674 (6.2323, 0.2633) -> (6.1716, 0.0877)
  line L675 (6.1716, 0.0877) -> (6.2513, -0.0947)
  line L676 (6.2513, -0.0947) -> (7.1918, -0.9262)
  line L677 (13.0608, -0.9276) -> (13.3259, -1.9933)
  line L678 (13.3259, -1.9933) -> (13.5397, -2.3755)
  line L679 (13.5397, -2.3755) -> (13.8151, -2.0986)
  line L680 (13.8151, -2.0986) -> (14.2649, -1.1868)
  line L681 (14.2649, -1.1868) -> (14.9242, 0.2595)
  line L682 (14.9242, 0.2595) -> (14.9423, 0.6152)
  line L683 (14.9423, 0.6152) -> (14.7683, 0.795)
  line L684 (14.7683, 0.795) -> (14.083, 1.0101)
  line L685 (14.083, 1.0101) -> (13.3656, 1.1865)
  line L686 (13.3656, 1.1865) -> (12.9676, 1.0954)
  line L687 (12.9676, 1.0954) -> (12.7751, 0.9875)
  line L688 (12.7751, 0.9875) -> (12.7207, 0.7408)
  line L689 (12.7207, 0.7408) -> (13.0608, -0.9276)
  line L690 (-1.2774, -0.0445) -> (-1.0413, -0.536)
  line L691 (-1.0413, -0.536) -> (-0.5208, -0.969)
  line L692 (-0.5208, -0.969) -> (0.0381, -1.2767)
  line L693 (0.0381, -1.2767) -> (0.5425, -0.8906)
  line L694 (0.5425, -0.8906) -> (0.9382, -0.3887)
  line L695 (0.9382, -0.3887) -> (0.7364, 0.1146)
  line L696 (0.7364, 0.1146) -> (0.5472, 0.4045)
  line L697 (0.5472, 0.4045) -> (0.3538, 0.5452)
  line L698 (0.3538, 0.5452) -> (-0.5156, 0.5375)
  line L699 (-0.5156, 0.5375) -> (-1.3237, 0.4043)
  line L700 (-1.3237, 0.4043) -> (-1.3716, 0.2466)
  line L701 (-1.3716, 0.2466) -> (-1.2774, -0.0445)
  line L702 (16.4568, -1.6448) -> (16.5625, -2.4896)
  line L703 (16.5625, -2.4896) -> (16.7839, -2.9235)
  line L704 (16.7839, -2.9235) -> (17.2884, -3.0833)
  line L705 (17.2884, -3.0833) -> (18.2436, -3.1062)
  line L706 (18.2436, -3.1062) -> (19.6861, -3.0237)
  line L707 (19.6861, -3.0237) -> (19.8664, -2.8278)
  line L708 (19.8664, -2.8278) -> (19.8922, -2.4462)
  line L709 (19.8922, -2.4462) -> (19.872, -2.0462)
  line L710 (19.872, -2.0462) -> (19.7302, -1.722)
  line L711 (19.7302, -1.722) -> (18.5957, -0.6135)
  line L712 (18.5957, -0.6135) -> (17.3396, 0.3693)
  line L713 (17.3396, 0.3693) -> (17.0551, 0.3872)
  line L714 (17.0551, 0.3872) -> (16.7717, 0.1897)
  line L715 (16.7717, 0.1897) -> (16.5118, -0.0489)
  line L716 (16.5118, -0.0489) -> (16.3923, -0.3195)
  line L717 (16.3923, -0.3195) -> (16.4568, -1.6448)
  line L718 (13.4614, -3.0009) -> (13.0181, -0.973)
  line L719 (13.0181, -0.973) -> (12.7426, 0.1239)
  line L720 (12.7426, 0.1239) -> (12.4879, 0.5912)
  line L721 (12.4879, 0.5912) -> (12.1074, 0.5204)
  line L722 (12.1074, 0.5204) -> (11.4547, 0.003)
  line L723 (11.4547, 0.003) -> (10.4383, -0.9607)
  line L724 (10.4383, -0.9607) -> (10.0256, -2.025)
  line L725 (10.0256, -2.025) -> (9.8744, -2.65)
  line L726 (9.8744, -2.65) -> (9.9865, -2.971)
  line L727 (9.9865, -2.971) -> (10.5083, -3.0892)
  line L728 (10.5083, -3.0892) -> (11.5859, -3.1061)
  line L729 (11.5859, -3.1061) -> (13.2247, -3.093)
  line L730 (13.2247, -3.093) -> (13.4614, -3.0009)
  line L731 (16.4043, -1.6474) -> (16.2089, -0.3339)
  line L732 (16.2089, -0.3339) -> (16.0164, -0.0859)
  line L733 (16.0164, -0.0859) -> (15.669, 0.1091)
  line L734 (15.669, 0.1091) -> (15.3115, 0.2555)
  line L735 (15.3115, 0.2555) -> (15.0491, 0.1631)
  line L736 (15.0491, 0.1631) -> (14.2939, -1.2464)
  line L737 (14.2939, -1.2464) -> (13.8646, -2.3216)
  line L738 (13.8646, -2.3216) -> (13.7978, -2.8737)
  line L739 (13.7978, -2.8737) -> (14.1622, -3.0771)
  line L740 (14.1622, -3.0771) -> (15.0267, -3.1062)
  line L741 (15.0267, -3.1062) -> (15.9012, -3.0835)
  line L742 (15.9012, -3.0835) -> (16.3363, -2.924)
  line L743 (16.3363, -2.924) -> (16.4612, -2.491)
  line L744 (16.4612, -2.491) -> (16.4043, -1.6474)
  line L745 (3.0414, -2.0181) -> (3.1757, -2.6471)
  line L746 (3.1757, -2.6471) -> (3.3336, -2.9701)
  line L747 (3.3336, -2.9701) -> (3.6169, -3.0891)
  line L748 (3.6169, -3.0891) -> (4.1274, -3.1061)
  line L749 (4.1274, -3.1061) -> (4.638, -3.0841)
  line L750 (4.638, -3.0841) -> (4.9219, -2.9297)
  line L751 (4.9219, -2.9297) -> (5.0815, -2.5106)
  line L752 (5.0815, -2.5106) -> (5.219, -1.6945)
  line L753 (5.219, -1.6945) -> (5.3372, -0.4251)
  line L754 (5.3372, -0.4251) -> (5.1966, -0.1895)
  line L755 (5.1966, -0.1895) -> (4.8804, -0.0092)
  line L756 (4.8804, -0.0092) -> (4.5492, 0.1396)
  line L757 (4.5492, 0.1396) -> (4.3033, 0.1555)
  line L758 (4.3033, 0.1555) -> (3.5802, -0.3329)
  line L759 (3.5802, -0.3329) -> (3.1513, -0.6952)
  line L760 (3.1513, -0.6952) -> (2.9522, -0.9915)
  line L761 (2.9522, -0.9915) -> (2.9324, -1.3798)
  line L762 (2.9324, -1.3798) -> (3.0414, -2.0181)
  line L763 (8.5563, -2.5081) -> (8.1866, -1.8687)
  line L764 (8.1866, -1.8687) -> (7.1771, -0.9814)
  line L765 (7.1771, -0.9814) -> (6.1644, -0.1834)
  line L766 (6.1644, -0.1834) -> (5.9569, -0.1165)
  line L767 (5.9569, -0.1165) -> (5.7729, -0.1696)
  line L768 (5.7729, -0.1696) -> (5.6031, -0.2592)
  line L769 (5.6031, -0.2592) -> (5.4942, -0.4481)
  line L770 (5.4942, -0.4481) -> (5.2711, -1.6963)
  line L771 (5.2711, -1.6963) -> (5.1769, -2.5113)
  line L772 (5.1769, -2.5113) -> (5.3191, -2.9299)
  line L773 (5.3191, -2.9299) -> (5.8542, -3.0841)
  line L774 (5.8542, -3.0841) -> (6.9383, -3.1061)
  line L775 (6.9383, -3.1061) -> (8.5512, -3.0314)
  line L776 (8.5512, -3.0314) -> (8.6789, -2.8539)
  line L777 (8.6789, -2.8539) -> (8.5563, -2.5081)
  point P0 (2.1873, -19.4723)
  constraints: 1556 end point, 17 parallel, 17 perpendicular
extrude "Extrusion7" cut sketch "Sketch12" along normal blind 4.15 and the other way blind 0.4 contours L407 L406 L405 L404 L403 L402 L401 L400 L399 L398 L397 L396 L395 L394 L393 L392 | L488 L487 L486 L485 L484 L483 L482 L481 L480 L479 L478 L477 L476 | L557 L556 L555 L554 L553 L552 L551 L550 L549 L548 L547 L546 L545 | L597 L596 L595 L594 L593 L592 L591 L590 L589 L588 L587 L586 L585 L584 L583 | L609 L608 L607 L606 L605 L604 L603 L602 L601 L600 L599 L598 | L623 L622 L621 L620 L619 L618 L617 L616 L615 L614 L613 L612 L611 L610 | L701 L700 L699 L698 L697 L696 L695 L694 L693 L692 L691 L690